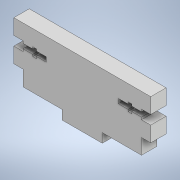
# Autodesk Inventor part: Крепление_мотора3_платформа
Saved by Autodesk Inventor 2020 (Build 240168000, 168)
## iProperties
Created: 2022-02-01
Part Number: Крепление_мотора3_платформа
Material: Типовые
Document SubType Name: Modeling
Designer: Администратор
Density: 1 g/cm^3
Appearance: По умолчанию
Autodesk Inventor part; units mm, degrees
ref_plane "YZ Plane" through (0, 0, 0) normal (1, 0, 0) x (0, 1, 0)
ref_plane "XZ Plane" through (0, 0, 0) normal (0, 1, 0) x (-1, 0, 0)
ref_plane "XY Plane" through (0, 0, 0) normal (0, 0, 1) x (1, 0, 0)
sketch "0" plane through (0, 0, 0) normal (0, 0, 1) x (1, 0, 0)
  line L0 (-44.5, -5) -> (-44.5, 5)
  line L1 (-44.5, 5) -> (-38.5, 5)
  line L2 (-38.5, 11) -> (-38.5, 9.5)
  line L3 (-38.5, 9.5) -> (-32.25, 9.5)
  line L4 (-23.5, 9.5) -> (-23.5, 6.5)
  line L5 (-23.5, 6.5) -> (-29.75, 6.5)
  line L6 (-32.25, 5.25) -> (-32.25, 6.5)
  line L7 (-32.25, 10.75) -> (-29.75, 10.75)
  line L8 (-29.75, 10.75) -> (-29.75, 9.5)
  line L9 (-29.75, 5.25) -> (-32.25, 5.25)
  line L10 (-32.25, 6.5) -> (-38.5, 6.5)
  line L11 (-29.75, 6.5) -> (-29.75, 5.25)
  line L12 (-32.25, 9.5) -> (-32.25, 10.75)
  line L13 (-38.5, 6.5) -> (-38.5, 5)
  line L14 (-44.5, 11) -> (-44.5, 21)
  line L15 (-38.5, 11) -> (-44.5, 11)
  line L16 (-44.5, 21) -> (-38.5, 21)
  line L17 (-29.75, 9.5) -> (-23.5, 9.5)
  line L18 (38.5, 21) -> (44.5, 21)
  line L19 (44.5, 21) -> (44.5, 11)
  line L20 (44.5, 11) -> (38.5, 11)
  line L21 (38.5, 5) -> (38.5, 6.5)
  line L22 (38.5, 6.5) -> (32.25, 6.5)
  line L23 (23.5, 6.5) -> (23.5, 9.5)
  line L24 (23.5, 9.5) -> (29.75, 9.5)
  line L25 (32.25, 10.75) -> (32.25, 9.5)
  line L26 (32.25, 5.25) -> (29.75, 5.25)
  line L27 (29.75, 5.25) -> (29.75, 6.5)
  line L28 (29.75, 10.75) -> (32.25, 10.75)
  line L29 (32.25, 9.5) -> (38.5, 9.5)
  line L30 (29.75, 9.5) -> (29.75, 10.75)
  line L31 (32.25, 6.5) -> (32.25, 5.25)
  line L32 (38.5, 9.5) -> (38.5, 11)
  line L33 (44.5, 5) -> (44.5, -5)
  line L34 (38.5, 5) -> (44.5, 5)
  line L35 (29.75, 6.5) -> (23.5, 6.5)
  line L36 (-38.5, 21) -> (38.5, 21)
  line L37 (38.5, -15) -> (13, -15)
  line L38 (13, -15) -> (13, -21)
  line L39 (-13, -21) -> (-13, -15)
  line L40 (-13, -15) -> (-38.5, -15)
  line L41 (-13, -21) -> (13, -21)
  line L42 (-44.5, -5) -> (-38.5, -5)
  line L43 (-38.5, -5) -> (-38.5, -15)
  line L44 (44.5, -5) -> (38.5, -5)
  line L45 (38.5, -5) -> (38.5, -15)
  constraints: 92 end point
sketch "Эскиз3" plane through (0, 0, 0) normal (0, 0, 1) x (1, 0, 0)
  line L0 (-44.5, 21) -> (-38.5, 21) projected
  line L1 (-38.5, 21) -> (38.5, 21) projected
  line L2 (38.5, 21) -> (44.5, 21) projected
  line L3 (44.5, 21) -> (44.5, 11) projected
  line L4 (44.5, 11) -> (38.5, 11) projected
  line L5 (38.5, 5) -> (44.5, 5) projected
  line L6 (38.5, 5) -> (38.5, 6.5) projected
  line L7 (38.5, 9.5) -> (38.5, 11) projected
  line L8 (32.25, 9.5) -> (38.5, 9.5) projected
  line L9 (38.5, 6.5) -> (32.25, 6.5) projected
  line L10 (32.25, 6.5) -> (32.25, 5.25) projected
  line L11 (32.25, 5.25) -> (29.75, 5.25) projected
  line L12 (29.75, 5.25) -> (29.75, 6.5) projected
  line L13 (29.75, 10.75) -> (32.25, 10.75) projected
  line L14 (32.25, 10.75) -> (32.25, 9.5) projected
  line L15 (29.75, 9.5) -> (29.75, 10.75) projected
  line L16 (29.75, 6.5) -> (23.5, 6.5) projected
  line L17 (23.5, 9.5) -> (29.75, 9.5) projected
  line L18 (23.5, 6.5) -> (23.5, 9.5) projected
  line L19 (44.5, 5) -> (44.5, -5) projected
  line L20 (44.5, -5) -> (38.5, -5) projected
  line L21 (38.5, -5) -> (38.5, -15) projected
  line L22 (13, -15) -> (13, -21) projected
  line L23 (38.5, -15) -> (13, -15) projected
  line L24 (-13, -21) -> (13, -21) projected
  line L25 (-13, -21) -> (-13, -15) projected
  line L26 (-13, -15) -> (-38.5, -15) projected
  line L27 (-38.5, -5) -> (-38.5, -15) projected
  line L28 (-44.5, -5) -> (-38.5, -5) projected
  line L29 (-44.5, -5) -> (-44.5, 5) projected
  line L30 (-44.5, 5) -> (-38.5, 5) projected
  line L31 (-38.5, 6.5) -> (-38.5, 5) projected
  line L32 (-32.25, 6.5) -> (-38.5, 6.5) projected
  line L33 (-32.25, 5.25) -> (-32.25, 6.5) projected
  line L34 (-29.75, 5.25) -> (-32.25, 5.25) projected
  line L35 (-29.75, 6.5) -> (-29.75, 5.25) projected
  line L36 (-23.5, 6.5) -> (-29.75, 6.5) projected
  line L37 (-23.5, 9.5) -> (-23.5, 6.5) projected
  line L38 (-29.75, 9.5) -> (-23.5, 9.5) projected
  line L39 (-29.75, 10.75) -> (-29.75, 9.5) projected
  line L40 (-32.25, 10.75) -> (-29.75, 10.75) projected
  line L41 (-32.25, 9.5) -> (-32.25, 10.75) projected
  line L42 (-38.5, 9.5) -> (-32.25, 9.5) projected
  line L43 (-38.5, 11) -> (-38.5, 9.5) projected
  line L44 (-38.5, 11) -> (-44.5, 11) projected
  line L45 (-44.5, 11) -> (-44.5, 21) projected
  line L46 (-44.5, 21) -> (44.5, 21)
  line L47 (44.5, 21) -> (44.5, 11)
  line L48 (-44.5, 11) -> (-44.5, 21)
  line L49 (23.5, 6.5) -> (23.5, 9.5)
  line L50 (29.75, 10.75) -> (32.25, 10.75)
  line L51 (32.25, 5.25) -> (29.75, 5.25)
  line L52 (44.5, 5) -> (38.5, 5)
  line L53 (44.5, 5) -> (38.5, 5)
  line L54 (38.5, -5) -> (44.5, -5)
  line L55 (44.5, -5) -> (44.5, 5)
  line L56 (13, -15) -> (38.5, -15)
  line L57 (38.5, -15) -> (38.5, -5)
  line L58 (13, -21) -> (-13, -21)
  line L59 (-13, -21) -> (-13, -15)
  line L60 (13, -15) -> (13, -21)
  line L61 (-13, -15) -> (-38.5, -15)
  line L62 (-38.5, -15) -> (-38.5, -5)
  line L63 (-44.5, 5) -> (-38.5, 5)
  line L64 (-38.5, -5) -> (-44.5, -5)
  line L65 (-44.5, -5) -> (-44.5, 5)
  line L66 (-44.5, 5) -> (-38.5, 5)
  line L67 (-23.5, 9.5) -> (-23.5, 6.5)
  line L68 (-32.25, 10.75) -> (-29.75, 10.75)
  line L69 (-29.75, 5.25) -> (-32.25, 5.25)
  line L70 (-32.25, 5.25) -> (-32.25, 6.5)
  line L71 (-32.25, 9.5) -> (-32.25, 10.75)
  line L72 (-29.75, 10.75) -> (-29.75, 9.5)
  line L73 (-29.75, 6.5) -> (-29.75, 5.25)
  line L74 (-38.5, 9.5) -> (-32.25, 9.5)
  line L75 (-29.75, 9.5) -> (-23.5, 9.5)
  line L76 (-23.5, 6.5) -> (-29.75, 6.5)
  line L77 (-32.25, 6.5) -> (-38.5, 6.5)
  line L78 (29.75, 5.25) -> (29.75, 6.5)
  line L79 (29.75, 9.5) -> (29.75, 10.75)
  line L80 (32.25, 10.75) -> (32.25, 9.5)
  line L81 (32.25, 6.5) -> (32.25, 5.25)
  line L82 (23.5, 9.5) -> (29.75, 9.5)
  line L83 (32.25, 9.5) -> (38.5, 9.5)
  line L84 (38.5, 6.5) -> (32.25, 6.5)
  line L85 (29.75, 6.5) -> (23.5, 6.5)
  line L86 (38.5, 5) -> (38.5, 6.5)
  line L87 (38.5, 9.5) -> (38.5, 11)
  line L88 (-38.5, 5) -> (-38.5, 6.5)
  line L89 (-38.5, 9.5) -> (-38.5, 11)
  line L90 (44.5, 11) -> (38.5, 11)
  line L91 (-38.5, 11) -> (-44.5, 11)
  line L92 (-44.5, 11) -> (-44.5, 10.75)
  line L93 (-44.5, 5.25) -> (-44.5, 5)
  line L94 (44.5, 11) -> (44.5, 10.75)
  line L95 (44.5, 5.25) -> (44.5, 5)
  point P0 (0, 0)
  constraints: 111 end point, 32 parallel, 10 horizontal, 8 perpendicular, 4 point on line
extrude "Выдавливание2" add sketch "0" along normal blind 10
